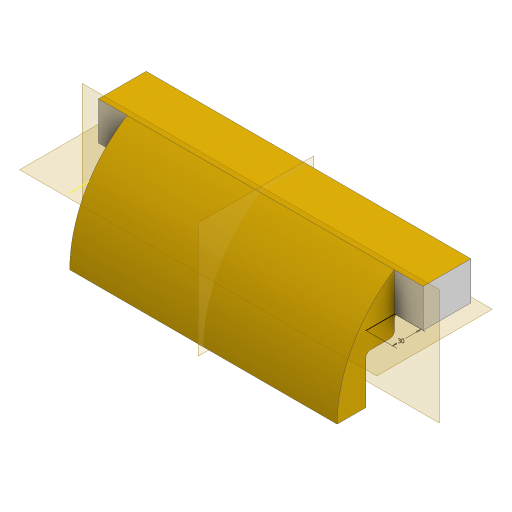
# Autodesk Inventor part: Крышка
Saved by Autodesk Inventor 2023.2 (Build 272271030, 271C)
## iProperties
Created: 2025-04-26
Part Number: Крышка
Material: Типовые
Document SubType Name: Modeling
Designer: Олег Коноваленко
Density: 1 g/cm^3
Appearance: По умолчанию
Author: Олег Коноваленко
Autodesk Inventor part; units mm, degrees
sketch "Эскиз1" plane through (0, 0, 0) normal (1, 0, 0) x (0, 1, 0)
  line L0 (-70, 60) -> (-70, 0)
  line L1 (-70, 0) -> (0, 0)
  line L2 (0, 0) -> (0, -50)
  line L3 (0, -50) -> (40, -50)
  line L4 (40, -50) -> (40, 0)
  arc A0 (40, 0) -> (-70, 60) centre (-69.545, -69.9992) ccw
  line L5 (0, 102.9525) -> (0, -98.8245) construction
  line L6 (-93.5412, 0) -> (71.2469, 0) construction
  dimension "d0" = 60
  dimension "d1" = 70
  dimension "d2" = 40
  dimension "d3" = 50
  dimension "d4" = 50
  dimension "d5" = 130
  constraints: 10 end point, 3 perpendicular, 2 point on circle, 2 point on line, 2 vertical, 1 centre point
  measures "d0" distance of L0.start L0.end
  measures "d1" distance of L0.end L1.end
  measures "d2" distance between parallel lines of L2 L4
  measures "d3" distance of L1.end L2.end
  measures "d4" distance of L3.end L4.end
  measures "d5" radius of A0
extrude "Выдавливание1" add sketch "Эскиз1" along normal mid plane 280
sketch "Эскиз2" plane through (-140, 0, 0) normal (0, -1, 0) x (1, 0, 0)
  line L0 (280, 0) -> (280, -50) projected
  line L1 (0, 60) -> (0, 0) projected
  line L2 (280, 0) -> (0, 0)
  line L3 (0, 0) -> (0, 30)
  line L4 (0, 30) -> (280, 30)
  line L5 (280, 30) -> (280, 0)
  point P0 (0, 0)
  dimension "d16" = 30
  constraints: 8 end point, 2 parallel, 1 horizontal, 1 midpoint, 1 perpendicular
  measures "d16" distance of L4.end L0.start
extrude "Выдавливание2" cut sketch "Эскиз2" along normal through all
extrude "Выдавливание3" add sketch "Эскиз2" along normal blind 20
fillet "Сопряжение2" radius 5 3 edges at (0, -20, 30) (0, 0, 0) (0, -20, 0)
sketch "Эскиз4" plane through (140, 0, 0) normal (1, 0, 0) x (0, 0, -1)
  line L0 (50, 0) -> (5, 0) projected
  arc A0 (0, 40) -> (-60, -70) centre (69.9992, -69.545) ccw projected
  line L1 (50, 0) -> (0, 0)
  line L2 (0, 0) -> (0, 40)
  line L3 (0, 40) -> (50, 40)
  line L4 (50, 40) -> (50, 0)
  point P0 (0, 0)
  point P1 (5, 0)
  constraints: 8 end point, 2 parallel, 1 horizontal, 1 perpendicular
extrude "Выдавливание4" add sketch "Эскиз4" along normal blind 30
mirror "Зеркальное отражение1" about plane through (0, 0, 0) normal (1, 0, 0) of "Выдавливание4"
